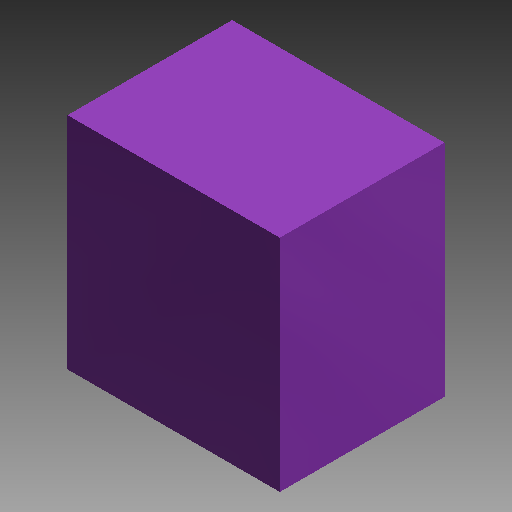
# Autodesk Inventor part: XAL5050-153MED
Saved by Autodesk Inventor 2018.2 (Build 222227000, 227)
## iProperties
Part Number: XAL5050-153MED
Material: Generic
Document SubType Name: Modeling
Designer: autocad
Appearance: XAL50XX-153, XAL5050-153MED
Author: autocad
Autodesk Inventor part; units mm, degrees
ref_plane "YZ Plane" through (0, 0, 0) normal (1, 0, 0) x (0, 1, 0)
ref_plane "XZ Plane" through (0, 0, 0) normal (0, 1, 0) x (-1, 0, 0)
ref_plane "XY Plane" through (0, 0, 0) normal (0, 0, 1) x (1, 0, 0)
sketch "XAL50XX-153, XAL5050-153MED_59" plane through (0, 0, 0) normal (0, 0, 1) x (1, 0, 0)
  line L0 (2.74, 2.84) -> (2.74, -2.84)
  line L1 (2.74, -2.84) -> (-2.74, -2.84)
  line L2 (-2.74, -2.84) -> (-2.74, 2.84)
  line L3 (-2.74, 2.84) -> (2.74, 2.84)
  constraints: 8 end point
extrude "Extrusion1" add sketch "XAL50XX-153, XAL5050-153MED_59" along normal blind 4.25
body "Solid1"
